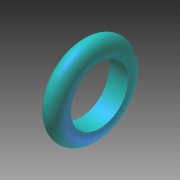
# Autodesk Inventor part: blue wheel tread
Saved by Autodesk Inventor 2012 (Build 160160000, 160)
## iProperties
Created: 2013-10-11
Part Number: blue wheel tread
Material: Default
Document SubType Name: Modeling
Designer: Bryce
Density: 1 g/cm^3
Author: Bryce
Autodesk Inventor part; units mm, degrees
ref_plane "YZ Plane" through (0, 0, 0) normal (1, 0, 0) x (0, 1, 0)
ref_plane "XZ Plane" through (0, 0, 0) normal (0, 1, 0) x (-1, 0, 0)
ref_plane "XY Plane" through (0, 0, 0) normal (0, 0, 1) x (1, 0, 0)
sketch "Sketch1" plane through (0, 0, 0) normal (0, 0, 1) x (1, 0, 0)
  line L0 (0, 0) -> (19.05, 0) construction
  line L1 (0, 28.575) -> (19.05, 28.575)
  line L2 (19.05, 28.575) -> (19.05, 31.75)
  line L3 (19.05, 31.75) -> (0, 31.75) construction
  line L4 (0, 31.75) -> (0, 28.575)
  ellipse E0 centre (9.525, 31.75) end of major axis (0, 31.75) minor radius 12.7 (19.05, 31.75) -> (0, 31.75) ccw
  point P0 (9.525, 44.45)
  dimension "d0" = 3.175
  dimension "d1" = 19.05
  dimension "d2" = 28.575
  dimension "d3" = 12.7
  dimension "d4" = 9.525
  dimension "d5" = 19.05
  constraints: 10 end point, 3 horizontal, 2 parallel, 1 midpoint, 1 perpendicular, 1 vertical alignment, 5 other
  measures "d0" distance of L3.end L1.start
  measures "d1" distance of L1.start L1.end
  measures "d2" distance from line of L0.start L1
  measures "d3" distance of point (9.525, 31.75) point (9.525, 44.45)
  measures "d4" distance from line of point (9.525, 44.45) L4
  measures "d5" distance of L0.start L0.end
revolve "Revolution1" add sketch "Sketch1" angle 360 about axis through (0, 0, 0) along (1, 0, 0)
equation "\"d4\" = 0.5 * d1"
equation "\"d5\" = d1"
body "Solid1"
